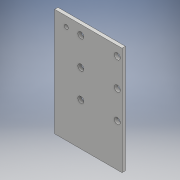
# Autodesk Inventor part: HeaderWheelSupport
Saved by Autodesk Inventor 2017 (Build 210142000, 142)
## iProperties
Created: 2016-12-11
Part Number: HeaderWheelSupport
Material: Generic
Document SubType Name: Modeling
Designer: umr
Density: 1 g/cm^3
Appearance: Default
Author: umr
Autodesk Inventor part; units mm, degrees
ref_plane "YZ Plane" through (0, 0, 0) normal (1, 0, 0) x (0, 1, 0)
ref_plane "XZ Plane" through (0, 0, 0) normal (0, 1, 0) x (-1, 0, 0)
ref_plane "XY Plane" through (0, 0, 0) normal (0, 0, 1) x (1, 0, 0)
sketch "Sketch1" plane through (0, 0, 0) normal (0, 1, 0) x (-1, 0, 0)
  line L0 (0, 0) -> (100, 0)
  line L1 (100, 0) -> (100, -110)
  line L2 (100, -110) -> (0, -110)
  line L3 (0, -110) -> (0, 0)
  dimension "d0" = 100
  dimension "d1" = 110
  constraints: 8 end point, 2 parallel, 1 horizontal, 1 perpendicular
  measures "d0" distance of L1.end L2.end
  measures "d1" distance of L0.end L1.end
extrude "Extrusion1" add sketch "Sketch1" along normal blind 5
sketch "Sketch2" plane through (0, 5, 0) normal (0, 1, 0) x (1, 0, 0)
  circle A0 centre (-7, 13.8333) radius 4.5
  line L0 (0, 0) -> (0, 110) projected
  line L1 (-100, 0) -> (0, 0) projected
  circle A1 centre (-7, 55.3333) radius 4.5
  circle A2 centre (-7, 96.8333) radius 4.5
  line L2 (-34, 0) -> (-34, 110)
  circle A3 centre (-61, 13.8333) radius 4.5
  circle A4 centre (-61, 55.3333) radius 4.5
  circle A5 centre (-61, 96.8333) radius 4.5
  circle A6 centre (-82.6974, 13.8333) radius 3
  dimension "d4" = 9
  dimension "d5" = 7
  dimension "d6" = 110
  dimension "d7" = 13.8333
  dimension "d10" = 41.5
  dimension "d19" = 27
  dimension "d20" = 6
  constraints: 7 centre point, 3 symmetric about line, 2 end point, 2 vertical, 1 point on line, 7 other
  measures "d4" diameter of A0
  measures "d5" distance from line of L0 A0.centre
  measures "d6" distance of L0.start L0.end
  measures "d7" distance from line of L1 A0.centre
  measures "d10" distance of A0.centre A1.centre
  measures "d19" distance from line of A2.centre L2
  measures "d20" diameter of A6
extrude "Extrusion2" cut sketch "Sketch2" against normal blind 10
sketch "Sketch3" plane through (0, 5, 0) normal (0, 1, 0) x (1, 0, 0)
  line L0 (-100, 110) -> (0, 110) projected
  line L1 (-100, 110) -> (0, 110)
  line L2 (0, 110) -> (0, 160)
  line L3 (0, 160) -> (-100, 160)
  line L4 (-100, 160) -> (-100, 110)
  point P0 (0, 0)
  dimension "d21" = 50
  constraints: 8 end point, 2 parallel, 1 horizontal, 1 perpendicular
  measures "d21" distance of L2.end L1.end
extrude "Extrusion3" add sketch "Sketch3" against normal blind 5
equation "\"d7\" = -0.5 * d4 + 0.166667 * d6"
equation "\"d10\" = -1.5 * d4 + 0.5 * d6"
body "Solid1"
